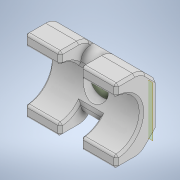
# Autodesk Inventor part: LargeCableHolderv2
Saved by Autodesk Inventor 2021 (Build 250183000, 183)
## iProperties
Created: 2021-02-22
Part Number: LargeCableHolderv2
Material: Generic
Document SubType Name: Modeling
Designer: Viktor
Density: 1 g/cm^3
Appearance: Default
Author: Viktor
## iProperties of the stored document _3DPrint.ipt
Created: 2021-02-22
Part Number: _3DPrint
Material: Generic
Document SubType Name: Modeling
Designer: Viktor
Density: 1 g/cm^3
Appearance: Default
Author: Viktor
Autodesk Inventor part; units mm, degrees
ref_plane "YZ Plane" through (0, 0, 0) normal (1, 0, 0) x (0, 1, 0)
ref_plane "XZ Plane" through (0, 0, 0) normal (0, 1, 0) x (-1, 0, 0)
ref_plane "XY Plane" through (0, 0, 0) normal (0, 0, 1) x (1, 0, 0)
sketch "Sketch1" plane through (0, 0, 0) normal (0, 0, 1) x (1, 0, 0)
  line L0 (-20, -16) -> (20, -16)
  line L1 (20, -16) -> (20, 16)
  line L2 (20, 16) -> (-20, 16)
  line L3 (-20, 16) -> (-20, -16)
  line L4 (-20, -16) -> (20, 16) construction
  line L5 (20, -16) -> (-20, 16) construction
  point P0 (0, 0)
  dimension "d0" = 32
  dimension "d1" = 40
  constraints: 12 end point, 2 midpoint, 2 parallel, 1 horizontal, 1 perpendicular
  measures "d0" distance between parallel lines of L0 L2
  measures "d1" distance between parallel lines of L1 L3
extrude "Extrusion1" add sketch "Sketch1" along normal blind 17
sketch "Sketch2" plane through (20, -16, 0) normal (1, 0, 0) x (0, 0, -1)
  line L0 (-33.6, 16) -> (5.6, 16) projected
  circle A0 centre (-17, 16) radius 11
  line L1 (0, 0) -> (0, 32) projected
  point P0 (0, 16)
  dimension "d4" = 22
  dimension "d5" = 6
  constraints: 1 centre point, 1 point on line
  measures "d4" diameter of A0
  measures "d5" distance edge to line of A0 L1
extrude "Extrusion2" cut sketch "Sketch2" against normal through all
chamfer "Chamfer1" distance 6 angle 45 2 edges at (0, 16, 0) (0, -16, 0)
fillet "Fillet1" radius 1 4 edges at (0, -11, 17) (0, 11, 17) (0, 16, 17) (0, -16, 17)
sketch "Sketch3" plane through (0, 0, 0) normal (0, 0, -1) x (-1, 0, 0)
  circle A0 centre (0, 0) radius 2.5
  dimension "d12" = 5
  constraints: 1 centre point, 1 coincident
  measures "d12" diameter of A0
extrude "Extrusion3" cut sketch "Sketch3" against normal through all
ref_plane "Work Plane1" through (0, 0, 3) normal (0, 0, -1) x (-1, 0, 0)
sketch "Sketch4" plane through (0, 0, 3) normal (0, 0, -1) x (-1, 0, 0)
  spline S0 degree 2 poles (2.5, 0) (2.5, 4.3301) (-1.25, 2.1651) (-5, 0) (-1.25, -2.1651) (2.5, -4.3301) (2.5, 0) knots 0 0 0 0.333333 0.333333 0.666667 0.666667 1 1 1 weights 1 0.5 1 0.5 1 0.5 1 projected
  spline S1 degree 5 poles (5.5, 0) (5.4989, 1.7696) (4.792, 3.5428) (3.3541, 4.9227) (-0.1528, 6.1742) (-3.5559, 4.7233) (-4.8567, 3.3718) (-6.1429, 0) (-4.8567, -3.3718) (-3.5559, -4.7233) (-0.1528, -6.1742) (3.3541, -4.9227) (4.792, -3.5428) (5.4989, -1.7696) (5.5, 0) knots 0 0 0 0 0 0 0.256119 0.256119 0.256119 0.5 0.5 0.5 0.743881 0.743881 0.743881 1 1 1 1 1 1
  point P0 (0, 0)
  dimension "d16" = 3
  constraints: 3 other
extrude "Extrusion4" cut sketch "Sketch4" against normal blind 15
sketch "Sketch6" plane through (-20, -16, 6) normal (0, -1, 0) x (1, 0, 0)
  line L0 (20, 14.4) -> (20, -9.4) projected
  line L1 (15.5, 2) -> (24.5, 2)
  line L2 (24.5, 2) -> (24.5, 11)
  line L3 (24.5, 11) -> (15.5, 11)
  line L4 (15.5, 11) -> (15.5, 2)
  line L5 (15.5, 2) -> (24.5, 11) construction
  line L6 (24.5, 2) -> (15.5, 11) construction
  line L7 (40, 11) -> (0, 11) projected
  point P0 (20, -6)
  point P1 (20, 6.5)
  point P2 (20, 11)
  dimension "d19" = 9
  dimension "d20" = 9
  constraints: 12 end point, 4 midpoint, 2 parallel, 1 horizontal, 1 perpendicular, 1 point on line
  measures "d19" distance between parallel lines of L2 L4
  measures "d20" distance between parallel lines of L3 L1
extrude "Extrusion5" cut sketch "Sketch6" against normal through all
fillet "Fillet3" radius 7 4 edges at (0, 16, 8) (0, -16, 8) (0, -16, 6) (0, 16, 6)
fillet "Fillet4" radius 4 2 edges at (0, -15.5425, 6.4105) (0, 15.5425, 6.4105)
chamfer "Chamfer2" distance 1 angle 45 54 edges at (-4.5, 15.4672, 6.2207) (-4.5, 12.5607, 2.5607) (-4.5, 16, 12.4497) (-4.5, 15.7071, 16.7071) (-4.5, 13.4791, 17) (-4.5, 11.2813, 16.736) (-4.5, 9.5414, 11.5263) (4.5, 16, 12.4497) (4.5, 15.7071, 16.7071) (4.5, 13.4791, 17) (4.5, 11.2813, 16.736) (4.5, 9.5414, 11.5263) (4.5, 15.4672, 6.2207) (4.5, 12.5607, 2.5607) (20, 16, 12.4497) (20, 15.7071, 16.7071) (20, 13.4791, 17) (20, 11.2813, 16.736) (20, 0, 6) (20, -11.2813, 16.736) (20, -13.4791, 17) (20, -15.7071, 16.7071) (20, -16, 12.4497) (20, -15.4672, 6.2207) (20, -11.9749, 1.9749) (20, 15.4672, 6.2207) (20, 11.9749, 1.9749) (-20, 16, 12.4497) (-20, 15.7071, 16.7071) (-20, 13.4791, 17) (-20, 11.2813, 16.736) (-20, 0, 6) (-20, -11.2813, 16.736) (-20, -13.4791, 17) (-20, -15.7071, 16.7071) (-20, -16, 12.4497) (-20, -15.4672, 6.2207) (-20, -11.9749, 1.9749) (-20, 15.4672, 6.2207) (-20, 11.9749, 1.9749) (-4.5, -16, 12.4497) (-4.5, -15.7071, 16.7071) (-4.5, -13.4791, 17) (-4.5, -11.2813, 16.736) (-4.5, -9.5414, 11.5263) (-4.5, -15.4672, 6.2207) (-4.5, -12.5607, 2.5607) (4.5, -16, 12.4497) (4.5, -15.4672, 6.2207) (4.5, -12.5607, 2.5607) (4.5, -15.7071, 16.7071) (4.5, -13.4791, 17) (4.5, -11.2813, 16.736) (4.5, -9.5414, 11.5263)
body "Solid1"
